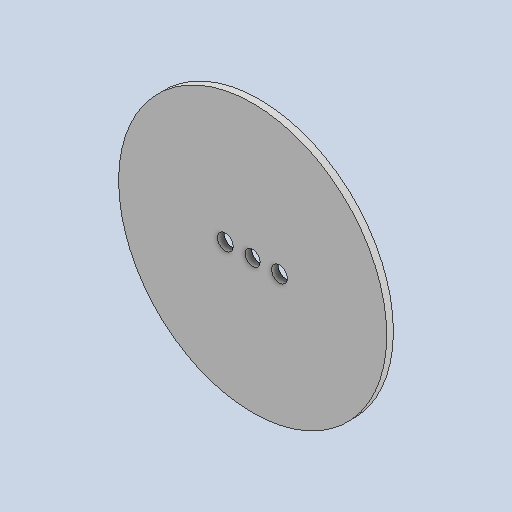
# Autodesk Inventor part: лицо1
Saved by Autodesk Inventor 2023.1 (Build 271208000, 208)
## iProperties
Created: 2024-12-06
Part Number: лицо1
Material: Типовые
Document SubType Name: Modeling
Designer: DELL
Density: 1 g/cm^3
Appearance: По умолчанию
Author: DELL
Autodesk Inventor part; units mm, degrees
ref_plane "YZ Plane" through (0, 0, 0) normal (1, 0, 0) x (0, 1, 0)
ref_plane "XZ Plane" through (0, 0, 0) normal (0, 1, 0) x (-1, 0, 0)
ref_plane "XY Plane" through (0, 0, 0) normal (0, 0, 1) x (1, 0, 0)
sketch "Эскиз1" plane through (0, 0, 0) normal (0, 0, 1) x (1, 0, 0)
  circle A0 centre (0, 0) radius 80 projected
  line L0 (-52.7251, -56.1362) -> (-52.7358, -38.0942) construction
  arc A1 (-51.7364, -37.0936) -> (-52.7358, -38.0942) centre (-51.7358, -38.0936) ccw construction
  line L1 (-51.7364, -37.0936) -> (-13.2571, -37.0709) construction
  arc A2 (-12.2565, -38.0703) -> (-13.2571, -37.0709) centre (-13.2565, -38.0709) ccw construction
  line L2 (-12.2565, -38.0703) -> (-12.2459, -56.1122) construction
  arc A3 (-13.2453, -57.1128) -> (-12.2459, -56.1122) centre (-13.2459, -56.1128) ccw construction
  line L3 (-13.2453, -57.1128) -> (-51.7245, -57.1356) construction
  arc A4 (-52.7251, -56.1362) -> (-51.7245, -57.1356) centre (-51.7251, -56.1356) ccw construction
  circle A5 centre (-11.4805, -27.7164) radius 3.15 construction
  circle A6 centre (-27.7164, 11.4805) radius 3.15 construction
  circle A7 centre (11.4805, 27.7164) radius 3.15 construction
  circle A8 centre (27.7164, -11.4805) radius 3.15 construction
  circle A9 centre (15.9974, -0.2901) radius 4.75 projected
  circle A10 centre (-16.284, 0.1089) radius 4.75 projected
  circle A11 centre (0, 0) radius 4.5 projected
  circle A12 centre (0, 0) radius 39.5 construction
  point P0 (0, 0)
extrude "Выдавливание1" add sketch "Эскиз1" along normal blind 4
